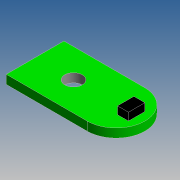
# Autodesk Inventor part: FE015
Saved by Autodesk Inventor 2015 SP1 (Build 190203100, 203)
## iProperties
Created: 2014-10-07
Part Number: FE015
Material: Fourniture / Geliefertes
Document SubType Name: Modeling
Designer: grp
Density: 1 g/cm^3
Appearance: Par défaut
Description: Capteur effet Hall
Author: grp
Autodesk Inventor part; units mm, degrees
ref_plane "YZ Plane" through (0, 0, 0) normal (1, 0, 0) x (0, 1, 0)
ref_plane "XZ Plane" through (0, 0, 0) normal (0, 1, 0) x (-1, 0, 0)
ref_plane "XY Plane" through (0, 0, 0) normal (0, 0, 1) x (1, 0, 0)
sketch "Sketch1" plane through (0, 0, 0) normal (0, 0, 1) x (1, 0, 0)
  line L0 (0, 0) -> (14.75, 0)
  arc A0 (14.75, 0) -> (14.75, 10.5) centre (14.75, 5.25) ccw
  line L1 (14.75, 10.5) -> (0, 10.5)
  line L2 (0, 10.5) -> (0, 0)
  dimension "d0" = 10.5
  dimension "d1" = 20
  constraints: 6 end point, 2 point on circle, 2 tangent, 1 centre point, 1 horizontal, 1 parallel, 1 perpendicular
  measures "d0" distance between parallel lines of L1 L0
extrude "Extrusion1" add sketch "Sketch1" along normal blind 1.6
sketch "Esquisse2" plane through (0, 0, 1.6) normal (0, 0, 1) x (1, 0, 0)
  line L0 (0, 0) -> (14.75, 0) construction
  arc A0 (14.75, 0) -> (14.75, 10.5) centre (14.75, 5.25) ccw construction
  line L1 (14.75, 10.5) -> (0, 10.5) construction
  line L2 (0, 10.5) -> (0, 0) construction
  line L3 (16.5, 6.75) -> (18.5, 6.75)
  line L4 (18.5, 6.75) -> (18.5, 3.75)
  line L5 (18.5, 3.75) -> (16.5, 3.75)
  line L6 (16.5, 3.75) -> (16.5, 6.75)
  point P0 (16.5, 5.25)
  dimension "d4" = 3
  dimension "d5" = 2
  dimension "d6" = 18.5
  constraints: 8 end point, 2 parallel, 1 horizontal, 1 horizontal alignment, 1 midpoint, 1 perpendicular
  measures "d4" distance of L3.end L4.end
  measures "d5" distance of L3.start L3.end
  measures "d6" distance between parallel lines of L2 L4
extrude "Extrusion2" add sketch "Esquisse2" along normal blind 1.4
sketch "Esquisse3" plane through (0, 0, 1.6) normal (0, 0, 1) x (1, 0, 0)
  line L0 (18.5, 6.75) -> (18.5, 3.75) construction
  line L1 (18.5, 3.75) -> (16.5, 3.75) construction
  line L2 (16.5, 3.75) -> (16.5, 6.75) construction
  line L3 (16.5, 6.75) -> (18.5, 6.75) construction
  line L4 (0, 0) -> (14.75, 0) construction
  arc A0 (14.75, 0) -> (14.75, 10.5) centre (14.75, 5.25) ccw construction
  line L5 (14.75, 10.5) -> (0, 10.5) construction
  line L6 (0, 10.5) -> (0, 0) construction
  line L7 (0, 5.25) -> (14.75, 5.25) construction
  point P0 (7, 5.25)
  dimension "d9" = 7
  constraints: 2 end point, 1 horizontal, 1 midpoint, 1 point on line
  measures "d9" distance from line of L6 point (7, 5.25)
hole "Perçage1" at (7, 5.25, 1.6) direction (0, 0, -1) diameter 3.2 end through all
